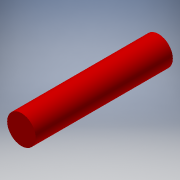
# Autodesk Inventor part: Front Noodle 2
Saved by Autodesk Inventor 2018 (Build 220112000, 112)
## iProperties
Created: 2018-01-17
Part Number: Front Noodle 2
Material: Generic
Document SubType Name: Modeling
Designer: Apple
Density: 1 g/cm^3
Appearance: Default
Author: Apple
Autodesk Inventor part; units mm, degrees
ref_plane "YZ Plane" through (0, 0, 0) normal (1, 0, 0) x (0, 1, 0)
ref_plane "XZ Plane" through (0, 0, 0) normal (0, 1, 0) x (-1, 0, 0)
sketch "Sketch1" plane through (0, 0, 0) normal (0, 0, 1) x (1, 0, 0)
  line L0 (0, 19.05) -> (127, 19.05) projected
  line L1 (127, 0) -> (127, 19.05) projected
  line L2 (127, 0) -> (127, 86.3927) construction
  circle A0 centre (95.25, 50.8) radius 31.75
  point P0 (0, 0)
  dimension "d0" = 63.5
  constraints: 2 end point, 2 tangent, 1 centre point, 1 vertical
  measures "d0" diameter of A0
ref_plane "Work Plane1" through (0, 0, -304.8) normal (0, 0, -1) x (0, 1, 0)
extrude "Extrusion1" add sketch "Sketch1" against normal up to surface (304.8 mm away)
body "Solid1"
